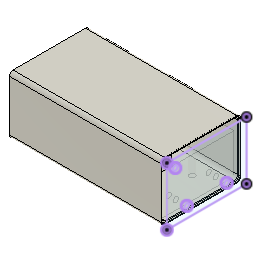
Juicebox (Autodesk Fusion 360 design; units mm, degrees)
Autodesk Fusion 360 part; units mm, degrees
note: some values were not read from the file. Set by a fixed rule: which face or edge a step refers to.
sketch "footprint" plane through (0, 0, 0) normal (0, 0, 1) x (1, 0, 0) in component "IP5328P"
  line L0 (0, 0) -> (65, 0)
  line L1 (65, 0) -> (65, 32.5)
  line L2 (65, 32.5) -> (0, 32.5)
  line L3 (0, 32.5) -> (0, 0)
  line L4 (32.5, 32.5) -> (32.5, 0) construction
  line L5 (65, 16.25) -> (0, 16.25) construction
  line L6 (62.5, 29.75) -> (2.5, 29.75) construction
  line L7 (2.5, 29.75) -> (2.5, 2.75) construction
  line L8 (2.5, 2.75) -> (62.5, 2.75) construction
  line L9 (62.5, 2.75) -> (62.5, 29.75) construction
  line L10 (62.5, 29.75) -> (2.5, 2.75) construction
  line L11 (2.5, 29.75) -> (62.5, 2.75) construction
  circle A0 centre (62.5, 29.75) radius 1.5
  circle A1 centre (62.5, 2.75) radius 1.5
  circle A2 centre (2.5, 2.75) radius 1.5
  circle A3 centre (2.5, 29.75) radius 1.5
  line L12 (8, 32.5) -> (21, 32.5)
  line L13 (21, 32.5) -> (21, 21.5)
  line L14 (21, 21.5) -> (8, 21.5)
  line L15 (8, 21.5) -> (8, 32.5)
  line L16 (28, 32.5) -> (37, 32.5)
  line L17 (37, 32.5) -> (37, 25.5)
  line L18 (37, 25.5) -> (28, 25.5)
  line L19 (28, 25.5) -> (28, 32.5)
  line L20 (44, 32.5) -> (57, 32.5)
  line L21 (57, 32.5) -> (57, 21.5)
  line L22 (57, 21.5) -> (44, 21.5)
  line L23 (44, 21.5) -> (44, 32.5)
  line L24 (0, 7) -> (7, 7)
  line L25 (7, 7) -> (7, 15)
  line L26 (7, 15) -> (0, 15)
  line L27 (0, 15) -> (0, 7)
  line L28 (0, 21) -> (4, 21)
  line L29 (4, 21) -> (4, 26)
  line L30 (4, 26) -> (0, 26)
  line L31 (0, 26) -> (0, 21)
  point P0 (32.5, 16.25)
  dimension "d1" = 65
  dimension "d2" = 32.5
  dimension "d5" = 60
  dimension "d6" = 27
  dimension "d7" = 3
  dimension "d8" = 3
  dimension "d9" = 3
  dimension "d10" = 3
  dimension "d11" = 13
  dimension "d12" = 11
  dimension "d13" = 8
  dimension "d14" = 9
  dimension "d15" = 7
  dimension "d16" = 7
  dimension "d17" = 8
  dimension "d27" = 7
  dimension "d28" = 8
  dimension "d29" = 7
  dimension "d30" = 4
  dimension "d31" = 5
  dimension "d32" = 6
  constraint horizontal L0
  constraint vertical L1
  constraint horizontal L2
  constraint vertical L3
  constraint coincident L0.start L3.end
  constraint midpoint L2 L4.start
  constraint perpendicular L2 L4
  constraint midpoint L1 L5.start
  constraint midpoint L3 L5.end
  constraint horizontal L6
  constraint perpendicular L6 L7
  constraint parallel L6 L8
  constraint parallel L7 L9
  constraint coincident L10 P0
  constraint coincident L11 P0
  constraint midpoint L5 P0
  constraint coincident L6.start L9.end
  constraint coincident L8.end L9.start
  constraint coincident L7.end L8.start
  constraint coincident L6.end L7.start
  constraint horizontal L12
  constraint vertical L13
  constraint horizontal L14
  constraint vertical L15
  constraint coincident L2 L12.start
  constraint horizontal L16
  constraint vertical L17
  constraint horizontal L18
  constraint vertical L19
  constraint coincident L2 L16.start
  constraint horizontal L20
  constraint vertical L21
  constraint horizontal L22
  constraint vertical L23
  constraint coincident L2 L20.start
  constraint equal L14 L22
  constraint equal L13 L23
  constraint horizontal L24
  constraint vertical L25
  constraint horizontal L26
  constraint vertical L27
  constraint coincident L3 L24.start
  constraint horizontal L28
  constraint vertical L29
  constraint horizontal L30
  constraint vertical L31
  constraint coincident L3 L28.start
  measures "d1" distance of L0.start L0.end
  measures "d2" distance of L0.start L2.end
  measures "d5" distance of L7.end L8.end
  measures "d6" distance of L6.end L7.end
  measures "d7" diameter of A0
  measures "d8" diameter of A1
  measures "d9" diameter of A2
  measures "d10" diameter of A3
  measures "d11" distance of L12.start L12.end
  measures "d12" distance of L12.start L14.end
  measures "d13" distance of L3 L15
  measures "d14" distance of L16.start L16.end
  measures "d15" distance of L16.start L18.end
  measures "d16" distance of L13 L19
  measures "d17" distance of L1 L21
  measures "d27" distance of L24.start L24.end
  measures "d28" distance of L24.start L26.end
  measures "d29" distance of L0 L24
  measures "d30" distance of L28.start L28.end
  measures "d31" distance of L28.start L30.end
  measures "d32" distance of L26 L28
extrude "Extrude1" add sketch "footprint" along normal blind 1.6 contours L0 L1 L2 L3 L13 L14 L15 L17 L18 L19 L21 L22 L23 L24 L25 L26 L28 L29 L30 | L3 L24 L25 L26 L27 | L3 L28 L29 L30 L31 | L2 L16 L17 L18 L19 makes body 1 in component "IP5328P"
extrude "Extrude2" add sketch "footprint" along normal blind 6 separate body contours L2 L20 L21 L22 L23 | L2 L12 L13 L14 L15 makes body 2 at (12.3333, 28.8333, 0) makes body 3 at (48.3333, 28.8333, 0) in component "IP5328P"
extrude "Extrude3" add sketch "footprint" along normal blind 4 from surface at 1.6 separate body contours L2 L16 L17 L18 L19 makes body 4 in component "IP5328P"
sketch "ports_front" plane through (0, 32.5, 0) normal (0, 1, 0) x (-1, 0, 0) in component "IP5328P"
  line L0 (-57, 0) -> (-44, 0)
  line L1 (-44, 0) -> (-44, 6)
  line L2 (-44, 6) -> (-57, 6)
  line L3 (-57, 6) -> (-57, 0)
  line L4 (-21, 0) -> (-8, 0)
  line L5 (-8, 0) -> (-8, 6)
  line L6 (-8, 6) -> (-21, 6)
  line L7 (-21, 6) -> (-21, 0)
  line L8 (-37, 1.6) -> (-28, 1.6)
  line L9 (-28, 1.6) -> (-28, 5.6)
  line L10 (-28, 5.6) -> (-37, 5.6)
  line L11 (-37, 5.6) -> (-37, 1.6)
  line L12 (-35, 1.6) -> (-30, 1.6)
  arc A0 (-30, 1.6) -> (-30, 5.6) centre (-30, 3.6) ccw
  line L13 (-30, 5.6) -> (-35, 5.6)
  arc A1 (-35, 5.6) -> (-35, 1.6) centre (-35, 3.6) ccw
  line L14 (-37, 3.6) -> (-28, 3.6) construction
  constraint tangent L12 A0
  constraint tangent A0 L13
  constraint parallel L12 L13
  constraint tangent L13 A1
  constraint tangent L12 A1
  constraint midpoint A1 L14.start
  constraint midpoint A0 L14.end
  constraint midpoint L9 L14.end
  constraint perpendicular L9 L14
  constraint midpoint L11 L14.start
  constraint collinear L10 L13
extrude "Extrude4" cut sketch "ports_front" against normal up to surface (7 mm away) contours L8 L10 L12 A0 L13 A1 keep common part bodies 4 in component "IP5328P"
extrude "Extrude5" add sketch "footprint" along normal blind 3 from surface at 1.6 separate body contours L3 L24 L25 L26 L27 makes body 5 in component "IP5328P"
extrude "Extrude6" add sketch "footprint" along normal blind 3.2 from surface at 1.6 separate body contours L3 L28 L29 L30 L31 makes body 6 in component "IP5328P"
sketch "ports_side" plane through (0, 0, 0) normal (-1, 0, 0) x (0, -1, 0) in component "IP5328P"
  line L0 (-26, 1.6) -> (-21, 1.6)
  line L1 (-21, 1.6) -> (-21, 4.8)
  line L2 (-21, 4.8) -> (-26, 4.8)
  line L3 (-26, 4.8) -> (-26, 1.6)
  circle A0 centre (-23.5, 3.2) radius 1
  line L4 (-26, 3.2) -> (-21, 3.2) construction
  line L5 (-23.5, 4.8) -> (-23.5, 1.6) construction
  line L6 (-15, 1.6) -> (-7, 1.6)
  line L7 (-7, 1.6) -> (-7, 4.6)
  line L8 (-7, 4.6) -> (-15, 4.6)
  line L9 (-15, 4.6) -> (-15, 1.6)
  line L10 (-15, 4.6) -> (-7, 4.6)
  line L11 (-15, 4.6) -> (-15, 3.4)
  line L12 (-13, 1.6) -> (-9, 1.6)
  line L13 (-13, 1.6) -> (-15, 3.4)
  line L14 (-7, 4.6) -> (-7, 3.4)
  line L15 (-15, 4.6) -> (-15, 3.4)
  line L16 (-7, 3.4) -> (-9, 1.6)
  dimension "d39" = 2
  dimension "d42" = 1.2
  dimension "d43" = 4
  constraint midpoint L3 L4.start
  constraint midpoint L1 L4.end
  constraint midpoint L2 L5.start
  constraint midpoint L0 L5.end
  constraint midpoint A0.centre L4
  constraint coincident L8 L9.start
  constraint coincident L7.end L8.start
  constraint perpendicular L7 L10
  constraint coincident L8.end L9.start
  constraint perpendicular L10 L11
  constraint coincident L6 L12.start
  constraint perpendicular L9 L12
  constraint midpoint L6 L12
  constraint coincident L7 L14.end
  constraint equal L14 L15
  measures "d39" diameter of A0
  measures "d42" distance of L8.end L11.end
  measures "d43" distance of L12.start L12.end
extrude "Extrude7" cut sketch "ports_side" against normal blind 1 contours L0 L1 L2 L3 bodies 6 in component "IP5328P"
extrude "Extrude8" cut sketch "ports_side" against normal blind 7 contours L6 L7 L8 L9 L10 L11 L12 L13 L14 L15 L16 | L6 L7 L16 keep common part bodies 5 in component "IP5328P"
sketch "Sketch1" plane through (0, 0, 0) normal (0, 0, 1) x (1, 0, 0) in component "Battery_Holder"
  line L0 (0, -9.5) -> (80, -9.5)
  line L1 (80, -9.5) -> (80, 32.5)
  line L2 (80, 32.5) -> (0, 32.5)
  line L3 (0, 32.5) -> (0, -9.5)
  line L4 (40, -9.5) -> (40, 32.5) construction
  line L5 (80, 11.5) -> (0, 11.5) construction
  line L6 (12, 1.5) -> (68, 1.5) construction
  line L7 (68, 1.5) -> (68, 21.5) construction
  line L8 (68, 21.5) -> (12, 21.5) construction
  line L9 (12, 21.5) -> (12, 1.5) construction
  line L10 (12, 1.5) -> (68, 21.5) construction
  line L11 (68, 1.5) -> (12, 21.5) construction
  circle A0 centre (68, 1.5) radius 1.5
  circle A1 centre (12, 1.5) radius 1.5
  circle A2 centre (12, 21.5) radius 1.5
  circle A3 centre (68, 21.5) radius 1.5
  line L12 (0, 0) -> (65, 0)
  line L13 (65, 0) -> (65, 32.5)
  line L14 (0, 32.5) -> (0, 0)
  line L15 (65, 32.5) -> (0, 32.5)
  point P0 (40, 11.5)
  point P1 (0, 32.5)
  dimension "d46" = 80
  dimension "d47" = 42
  dimension "d48" = 56
  dimension "d49" = 20
  dimension "d50" = 3
  dimension "d51" = 3
  dimension "d52" = 3
  dimension "d53" = 3
  constraint horizontal L0
  constraint vertical L1
  constraint horizontal L2
  constraint vertical L3
  constraint midpoint L0 L4.start
  constraint midpoint L2 L4.end
  constraint midpoint L1 L5.start
  constraint midpoint L3 L5.end
  constraint horizontal L6
  constraint perpendicular L6 L7
  constraint parallel L6 L8
  constraint parallel L7 L9
  constraint coincident L10 P0
  constraint coincident L11 P0
  constraint midpoint L5 P0
  constraint coincident L6.end L7.start
  constraint coincident L6.start L9.end
  constraint coincident L8.end L9.start
  constraint coincident L7.end L8.start
  constraint coincident P1 L2.end
  measures "d46" distance of L0.start L0.end
  measures "d47" distance of L0.start L2.end
  measures "d48" distance of L7.end L8.end
  measures "d49" distance of L6.end L7.end
  measures "d50" diameter of A0
  measures "d51" diameter of A1
  measures "d52" diameter of A2
  measures "d53" diameter of A3
extrude "Extrude1'" add sketch "Sketch1" against normal blind 22 from surface at -2 separate body makes body 7 in component "Battery_Holder"
sketch "Midplate" plane through (0, 0, 0) normal (0, 0, 1) x (1, 0, 0) in component "Enclosure"
  circle A0 centre (68, 21.5) radius 1.5
  circle A1 centre (12, 21.5) radius 1.5
  circle A2 centre (68, 1.5) radius 1.5
  circle A3 centre (12, 1.5) radius 1.5
  line L0 (80, 32.5) -> (0, 32.5)
  line L1 (0, 32.5) -> (0, -9.5)
  line L2 (0, -9.5) -> (80, -9.5)
  line L3 (80, -9.5) -> (80, 32.5)
  circle A4 centre (2.5, 2.75) radius 1.5
  circle A5 centre (62.5, 2.75) radius 1.5
  circle A6 centre (2.5, 29.75) radius 1.5
  circle A7 centre (62.5, 29.75) radius 1.5
  line L4 (44, 32.5) -> (21, 32.5)
  line L5 (21, 32.5) -> (21, 21.5)
  line L6 (21, 21.5) -> (8, 21.5)
  line L7 (8, 21.5) -> (8, 32.5)
  line L8 (8, 32.5) -> (0, 32.5)
  line L9 (0, 32.5) -> (0, 0)
  line L10 (0, 0) -> (65, 0)
  line L11 (65, 0) -> (65, 32.5)
  line L12 (65, 32.5) -> (57, 32.5)
  line L13 (57, 32.5) -> (57, 21.5)
  line L14 (57, 21.5) -> (44, 21.5)
  line L15 (44, 21.5) -> (44, 32.5)
  line L16 (62.5, 2.75) -> (62.5, 29.75) construction
  line L17 (68, 21.5) -> (12, 21.5) construction
  line L18 (12, 21.5) -> (12, 1.5) construction
  line L19 (12, 1.5) -> (62.5, 2.75) construction
  line L20 (68, 1.5) -> (62.5, 2.75) construction
  line L21 (12, 1.5) -> (2.5, 2.75) construction
  line L22 (2.5, 2.75) -> (2.5, 29.75) construction
  line L23 (2.5, 29.75) -> (12, 21.5) construction
  circle A8 centre (2.5, 29.75) radius 2.5
  circle A9 centre (2.5, 2.75) radius 2.5
  circle A10 centre (12, 1.5) radius 2.5
  circle A11 centre (62.5, 2.75) radius 2.5
  circle A12 centre (68, 1.5) radius 2.5
  circle A13 centre (68, 21.5) radius 2.5
  circle A14 centre (62.5, 29.75) radius 2.5
  circle A15 centre (12, 21.5) radius 2.5
  line L24 (61.5, 20.5) -> (13, 20.5)
  line L25 (13, 20.5) -> (13, 2.5251)
  line L26 (13, 2.5251) -> (61.5, 3.7256)
  line L27 (61.5, 3.7256) -> (61.5, 20.5)
  line L28 (11, 21.5) -> (11, 0.4749)
  line L29 (11, 0.4749) -> (63.5, 1.7744)
  line L30 (63.5, 1.7744) -> (63.5, 29.75)
  line L31 (68, 22.5) -> (12, 22.5)
  line L32 (68.2216, 2.4751) -> (62.7216, 3.7251)
  line L33 (67.7784, 0.5249) -> (62.2784, 1.7749)
  line L34 (12.1305, 2.4915) -> (3.5, 3.627)
  line L35 (3.5, 3.627) -> (3.5, 27.5571)
  line L36 (3.5, 27.5571) -> (11.3443, 20.745)
  line L37 (11.8695, 0.5085) -> (1.5, 1.873)
  line L38 (1.5, 1.873) -> (1.5, 31.9429)
  line L39 (1.5, 31.9429) -> (12.6557, 22.255)
  line L40 (61.5, 2.75) -> (61.5, 29.75)
  line L41 (68, 20.5) -> (12, 20.5)
  dimension "d57" = 1
  dimension "d58" = 1
  dimension "d59" = 1
  dimension "d60" = 1
  dimension "d61" = 1
  dimension "d62" = 1
  dimension "d63" = 1
  dimension "d64" = 1
  dimension "d65" = -1
  dimension "d66" = 1
  dimension "d67" = 1
  dimension "d68" = 1
  dimension "d69" = -1
  dimension "d70" = 1
  dimension "d71" = -1
  dimension "d72" = -1
  dimension "d75" = -1
  constraint coincident A5.centre L16.start
  constraint coincident A7.centre L16.end
  constraint coincident A0.centre L17.start
  constraint coincident A1.centre L17.end
  constraint coincident A3.centre L18.end
  constraint coincident A2.centre L20.start
  constraint coincident A4.centre L21.end
  constraint coincident A6.centre L22.end
extrude "Extrude1''" add sketch "Midplate" against normal up to surface (2 mm away) separate body contours A0 A13 L31 L41 | A0 A13 L31 L41 | L11 A13 L31 L41 | L11 L30 L31 L41 | A7 A14 L30 L40 | A14 L30 L31 L40 | L30 L31 L40 L41 | L11 A12 L32 L33 | L11 A11 L32 | A11 L27 L30 L40 L41 | A7 A14 L30 L40 | L5 L6 L13 L14 L15 A15 L24 L31 L40 L41 | A5 A11 L32 L33 | L11 A11 L33 | A2 A12 L32 L33 | A2 A12 L32 L33 | A5 A11 L30 L32 | A5 A11 L27 L30 L40 | L13 L14 L15 L31 | A5 A11 L29 L33 | A5 A11 L26 L27 L40 | A1 L6 A15 L24 L41 | A1 A15 L24 L25 L41 | A10 A11 L26 L29 | A5 A11 L26 L29 | A10 A15 L25 L28 | A1 A15 L25 L28 | L5 L6 A15 L31 | A1 L6 A15 L31 | L10 A10 | A3 L10 A10 L29 | A3 A10 L26 L29 | A3 A10 L25 L26 | A1 L6 A15 L28 L36 | A3 A10 L25 L28 L34 | A1 A15 L31 L39 | A3 L10 A10 L37 | L6 A15 L36 | A10 L28 L34 | A1 L6 A15 L36 L39 | L7 A15 L36 L39 | A4 A9 L37 L38 | L7 A8 L36 L39 | A3 A10 L28 L34 L37 | A9 A10 L34 L37 | A1 L6 L36 | A3 L28 L34 | A6 A8 L38 L39 | A8 A9 L35 L38 | A4 A9 L35 L38 | A4 A9 L34 L37 | A6 A8 L35 L36 L38 L39 | A4 A9 L34 L35 | A6 L38 L39 picked at (1.7525, 31.3892) makes body 8 in component "Enclosure"
sketch "Box_face" plane through (80, 0, 0) normal (1, 0, 0) x (0, 1, 0) in component "Enclosure"
  line L0 (32.5, -2) -> (-9.5, -2)
  line L1 (-9.5, -2) -> (-9.5, -24)
  line L2 (-9.5, -24) -> (32.5, -24)
  line L3 (32.5, -24) -> (32.5, -2)
  line L4 (21.5, 0) -> (32.5, 0)
  line L5 (32.5, 0) -> (32.5, 6)
  line L6 (32.5, 6) -> (21.5, 6)
  line L7 (21.5, 6) -> (21.5, 0)
  line L8 (32.5, 0) -> (32.5, -2)
  line L9 (-9.5, 6) -> (-9.5, -2)
  line L10 (-9.5, 6) -> (21.5, 6)
  constraint coincident L4.end L5.start
  constraint coincident L0.start L3.end
  constraint coincident L0.end L1.start
  constraint perpendicular L0 L9
  constraint coincident L6.end L7.start
  constraint collinear L6 L10
extrude "Extrude3'" add sketch "Box_face" against normal up to surface (82 mm away) from surface at 2 separate body makes body 9 in component "Enclosure"
shell "Shell2" thickness 1 outward yes removed faces 1 at (82, 14.8333, -14) on bodies 9 in component "Enclosure"
extrude "Extrude4'" cut sketch "ports_front" along normal through all contours L0 L1 L2 L3 | L4 L5 L6 L7 | L8 L10 L12 A0 L13 A1 bodies 9 in component "Enclosure"
extrude "Extrude5'" cut sketch "ports_side" along normal through all contours L0 L1 L2 L3 | A0 | L6 L7 L8 L9 L10 L11 L12 L13 L14 L15 L16 bodies 9 in component "Enclosure"
sketch "Case_backside" plane through (-1, 0, 0) normal (-1, 0, 0) x (0, -1, 0)
  line L0 (-13, 1.6) -> (-15, 3.4)
  line L1 (-15, 3.4) -> (-15, 4.6)
  line L2 (-15, 4.6) -> (-7, 4.6)
  line L3 (-7, 4.6) -> (-7, 3.4)
  line L4 (-9, 1.6) -> (-13, 1.6)
  line L5 (-21, 1.6) -> (-26, 1.6)
  line L6 (-26, 1.6) -> (-26, 4.8)
  line L7 (-26, 4.8) -> (-21, 4.8)
  line L8 (-21, 4.8) -> (-21, 1.6)
  line L9 (-33.5, -25) -> (10.5, -25)
  line L10 (10.5, -25) -> (10.5, 7)
  line L11 (10.5, 7) -> (-33.5, 7)
  line L12 (-33.5, 7) -> (-33.5, -25)
  circle A0 centre (-23.5, 3.2) radius 1
  circle A1 centre (-23.5, 3.2) radius 1
  line L13 (-26, 4.8) -> (-26, 1.6)
  line L14 (-26, 1.6) -> (-21, 1.6)
  line L15 (-21, 1.6) -> (-21, 4.8)
  line L16 (-21, 4.8) -> (-26, 4.8)
  circle A2 centre (-23.5, 3.2) radius 1.4
  line L17 (-22.9911, 4.8) -> (-22.9911, 1.6)
  line L18 (-23.5, 4.8) -> (-23.5, 1.6) construction
  line L19 (-24.0089, 4.8) -> (-24.0089, 1.6)
  line L20 (-7, 3.4) -> (-9, 1.6)
  dimension "d88" = 0.4
  constraint coincident L7 L17.start
  constraint coincident L5 L17.end
  constraint perpendicular L5 L17
  constraint midpoint L7 L18.start
  constraint midpoint L5 L18.end
  constraint symmetric L17.start L18 L19.start
  constraint symmetric L17.end L18 L19.end
extrude "Extrude6'" add sketch "Case_backside" against normal up to surface (1 mm away) contours L5 L14 A2 L17 L19 | A0 A1 A2 L17 | A0 A1 A2 L17 L19 | A0 A1 A2 L19 | A0 A1 L17 | A0 A1 L17 L19 | A0 A1 A2 L17 L19 | A0 A1 L19 bodies 9 in component "Enclosure"
sketch "Sketch2" plane through (80, 0, 0) normal (1, 0, 0) x (0, 1, 0) in component "Battery_Holder"
  line L0 (32.5, -2) -> (-9.5, -2)
  line L1 (-9.5, -2) -> (-9.5, -24)
  line L2 (-9.5, -24) -> (32.5, -24)
  line L3 (32.5, -24) -> (32.5, -2)
  line L4 (22.5, -24) -> (22.5, -19) construction
  line L5 (22.5, -19) -> (32.5, -19) construction
  circle A0 centre (22.5, -19) radius 1.25
  line L6 (11.5, -2) -> (11.5, -24)
  circle A1 centre (0.5, -19) radius 1.25
  dimension "d91" = 5
  dimension "d93" = 10
  dimension "d94" = 2.5
  constraint coincident L2 L4.start
  constraint perpendicular L2 L4
  constraint coincident L3 L5.end
  constraint perpendicular L3 L5
  constraint coincident L4.end L5.start
  constraint midpoint L0 L6.start
  constraint midpoint L2 L6.end
  constraint symmetric A0 L6 A1
  measures "d91" distance of L4.start L4.end
  measures "d93" distance of L4.end L5.end
  measures "d94" diameter of A0
sketch "Cover_face" plane through (82, 0, 0) normal (1, 0, 0) x (0, 1, 0) in component "Enclosure"
  line L0 (-9.5, 6) -> (32.5, 6)
  line L1 (32.5, 6) -> (32.5, -24)
  line L2 (32.5, -24) -> (-9.5, -24)
  line L3 (-9.5, -24) -> (-9.5, 6)
  line L4 (-10.5, 7) -> (-10.5, -25)
  line L5 (-10.5, -25) -> (33.5, -25)
  line L6 (33.5, -25) -> (33.5, 7)
  line L7 (33.5, 7) -> (-10.5, 7)
  circle A0 centre (22.5, -19) radius 1.25
  circle A1 centre (0.5, -19) radius 1.25
  line L8 (-3.9083, 6) -> (-3.9083, 2.3132)
  line L9 (-5.9083, 0.3132) -> (-9.5, 0.3132)
  circle A2 centre (-5.9083, 2.3132) radius 1.25
  arc A3 (-5.9083, 0.3132) -> (-3.9083, 2.3132) centre (-5.9083, 2.3132) ccw
  line L10 (-9.9, 6.4) -> (32.9, 6.4)
  line L11 (32.9, 6.4) -> (32.9, -24.4)
  line L12 (32.9, -24.4) -> (-9.9, -24.4)
  line L13 (-9.9, -24.4) -> (-9.9, 6.4)
  line L14 (33.1, -24.6) -> (-10.1, -24.6)
  line L15 (-10.1, -24.6) -> (-10.1, 6.6)
  line L16 (-10.1, 6.6) -> (33.1, 6.6)
  line L17 (33.1, 6.6) -> (33.1, -24.6)
  dimension "d98" = 2.5
  dimension "d99" = 2
  dimension "d100" = -0.4
  dimension "d107" = -0.6
  constraint coincident L0 L8.start
  constraint perpendicular L0 L8
  constraint coincident L3 L9.end
  constraint perpendicular L3 L9
  constraint tangent L8 A3
  constraint tangent L9 A3
  constraint coincident A2.centre A3.centre
  measures "d98" diameter of A2
  measures "d99" radius of A3
extrude "Extrude7'" add sketch "Cover_face" against normal blind 2 contours L0 L3 L8 L9 A3 bodies 9 in component "Enclosure"
extrude "Extrude8'" add sketch "Cover_face" along normal blind 4 separate body contours L0 L3 L8 L9 A3 | L0 L1 L2 L3 L8 L9 A3 | L4 L5 L6 L7 | L10 L11 L12 L13 | L14 L15 L16 L17 makes body 10 in component "Enclosure"
extrude "Extrude10" cut sketch "Cover_face" along normal blind 1.4 contours L4 L5 L6 L7 | L14 L15 L16 L17 bodies 10 in component "Enclosure"
extrude "Extrude9" add sketch "Cover_face" along normal blind 0.8 contours L4 L5 L6 L7 bodies 9 in component "Enclosure"
sketch "Screw_Bores" plane through (86, 0, 0) normal (1, 0, 0) x (0, 1, 0) in component "Enclosure"
  circle A0 centre (22.5, -19) radius 1.25
  circle A1 centre (-5.9083, 2.3132) radius 1.25
  circle A2 centre (0.5, -19) radius 1.25
  line L0 (33.5, 7) -> (-10.5, 7)
  line L1 (-10.5, 7) -> (-10.5, -25)
  line L2 (-10.5, -25) -> (33.5, -25)
  line L3 (33.5, -25) -> (33.5, 7)
  circle A3 centre (-5.9083, 2.3132) radius 1.25
  circle A4 centre (0.5, -19) radius 1.25
  circle A5 centre (22.5, -19) radius 1.25
  line L4 (-10.5, -25) -> (33.5, -25)
  line L5 (33.5, -25) -> (33.5, 7)
  line L6 (33.5, 7) -> (-10.5, 7)
hole "Hole1" at (86, -5.9083, 2.3132) at (86, 0.5, -19) at (86, 22.5, -19) direction (-1, 0, 0) diameter 2.9 depth 10 tip angle 180 counterbore diameter 5.5 counterbore depth 2.5 bodies 7 in component "Battery_Holder"
hole "Hole1'" at (86, -5.9083, 2.3132) at (86, 0.5, -19) at (86, 22.5, -19) direction (-1, 0, 0) diameter 2.9 depth 10 tip angle 180 counterbore diameter 5.5 counterbore depth 2.5 bodies 9 in component "Enclosure"
fillet "Fillet1" radius 2 19 edges at (40.9, 33.5, 7) (40.9, -10.5, 7) (40.9, 33.5, -25) (40.9, -10.5, -25) (82.4, -10.1, 6.6) (82.4, 33.1, 6.6) (69.5, 32.5, 6) (41, 32.5, -24) (82.4, 33.1, -24.6) (41, -9.5, -24) (82.4, -10.1, -24.6) (84.7, 33.5, 7) (84.7, -10.5, 7) (84.7, 33.5, -25) (84.7, -10.5, -25) (82.7, -9.9, 6.4) (82.7, -9.9, -24.4) (82.7, 32.9, 6.4) (82.7, 32.9, -24.4) on bodies 9 10 in component "Enclosure"
component "IP5328P" placed x (1, 0, 0) y (0, 1, 0) z (0, 0, 1) at (0, 0, 0)
component "Battery_Holder" placed x (1, 0, 0) y (0, 1, 0) z (0, 0, 1) at (0, 0, 0)
component "Enclosure" placed x (1, 0, 0) y (0, 1, 0) z (0, 0, 1) at (0, 0, 0)
hidden bodies 10
named bodies: "PCB", "USBA_2", "USBA_1", "USBC", "microUSB", "Button", "Midplate", "Case", "Case_Cap"
